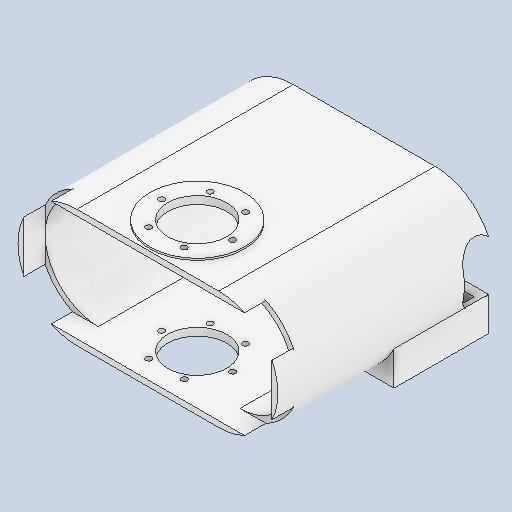
# Autodesk Inventor part: motor_holder_1
Saved by Autodesk Inventor 2025.3 (Build 293356030, 356C)
## iProperties
Created: 2025-09-06
Part Number: motor_holder_1
Material: PLA+ filament
Document SubType Name: Modeling
Designer: MSI
Density: 1.23 g/cm^3
Appearance: 일반
Mass: 781.424 g
Surface Area: 2127.56 cm^2
Volume: 635.304 cm^3
Author: MSI
Autodesk Inventor part; units mm, degrees
ref_plane "YZ Plane" through (0, 0, 0) normal (1, 0, 0) x (0, 1, 0)
ref_plane "XZ Plane" through (0, 0, 0) normal (0, 1, 0) x (-1, 0, 0)
ref_plane "XY Plane" through (0, 0, 0) normal (0, 0, 1) x (1, 0, 0)
sketch "스케치1" plane through (0, 0, 0) normal (0, 0, 1) x (1, 0, 0)
  circle A0 centre (-60, 0) radius 45
  circle A1 centre (60, 0) radius 45
  line L0 (-60, 45) -> (60, 45)
  line L1 (60, -45) -> (-60, -45)
  circle A2 centre (-60, 0) radius 50
  circle A3 centre (60, 0) radius 50
  line L2 (-60, 50) -> (60, 50)
  line L3 (60, -50) -> (-60, -50)
  point P0 (0, 0)
  point P1 (0, 45)
  dimension "d0" = 90
  dimension "d1" = 120
  dimension "d2" = 5
  constraints: 8 end point, 8 point on circle, 8 tangent, 4 centre point, 2 equal radius, 2 horizontal alignment, 1 midpoint, 1 vertical alignment
  measures "d0" diameter of A0
  measures "d1" distance of L1.start L1.end
  measures "d2" radial gap between concentric circles of A0 A2
extrude "돌출1" add sketch "스케치1" along normal mid plane 178 contours A0 L0 A2 L1 | A0 L1 A2 L0 | A2 L2 A3 L0 | L0 A3 L1 A2 | L1 A3 L3 A2 | A3 L1 A1 L0 | L0 A1 L1 A3
sketch "스케치2" plane through (0, 0, -89) normal (0, 0, -1) x (-1, 0, 0)
  arc A0 (-60, 50) -> (-60, -50) centre (-60, 0) ccw projected
  line L0 (-60, -50) -> (60, -50) projected
  arc A1 (60, -50) -> (60, 50) centre (60, 0) ccw projected
  line L1 (60, 50) -> (-60, 50) projected
  circle A2 centre (60, 0) radius 45 projected
  circle A3 centre (-60, 0) radius 45 projected
  point P0 (0, 0)
extrude "돌출2" add sketch "스케치2" along normal blind 5 contours L1 A1 L0 A0 | A2 | A3
sketch "스케치4" plane through (0, 0, 89) normal (0, 0, 1) x (1, 0, 0)
  line L0 (20, 15) -> (-20, 15)
  line L1 (-20, 15) -> (-20, -15)
  line L2 (-20, -15) -> (20, -15)
  line L3 (20, -15) -> (20, 15)
  line L4 (20, 15) -> (-20, -15) construction
  line L5 (-20, 15) -> (20, -15) construction
  point P0 (0, 0)
  dimension "d14" = 40
  dimension "d15" = 30
  constraints: 12 end point, 2 midpoint, 2 parallel, 1 horizontal, 1 perpendicular
  measures "d14" distance of L2.end L1.end
  measures "d15" distance of L1.end L0.end
extrude "돌출4" cut sketch "스케치4" against normal up to surface (178 mm away)
sketch "스케치5" plane through (0, 0, 89) normal (0, 0, 1) x (1, 0, 0)
  arc A0 (17.5736, -15) -> (17.5736, 15) centre (60, 0) ccw projected
  line L0 (-60, 45) -> (60, 45)
  line L1 (60, 45) -> (60, -45)
  line L2 (60, -45) -> (-60, -45)
  line L3 (-60, -45) -> (-60, 45)
  line L4 (-60, 45) -> (60, -45) construction
  line L5 (60, 45) -> (-60, -45) construction
  point P0 (0, 0)
  constraints: 12 end point, 2 midpoint, 2 parallel, 2 tangent, 1 horizontal, 1 perpendicular, 1 point on circle
extrude "돌출5" cut sketch "스케치5" against normal blind 150 contours L2 L3 L0 L1
sketch "스케치6" plane through (0, 0, 89) normal (0, 0, 1) x (1, 0, 0)
  line L0 (105, 45) -> (-105, 45)
  line L1 (-105, 45) -> (-105, -45)
  line L2 (-105, -45) -> (105, -45)
  line L3 (105, -45) -> (105, 45)
  line L4 (105, 45) -> (-105, -45) construction
  line L5 (-105, 45) -> (105, -45) construction
  line L6 (-60, 45) -> (60, 45) projected
  arc A0 (-60, 45) -> (-60, -45) centre (-60, 0) ccw projected
  point P0 (0, 0)
  constraints: 12 end point, 2 midpoint, 2 parallel, 1 collinear, 1 horizontal, 1 perpendicular, 1 tangent
extrude "돌출6" cut sketch "스케치6" against normal blind 18
sketch "스케치3" plane through (0, 0, 0) normal (1, 0, 0) x (0, 1, 0)
  line L0 (10, -84) -> (-10, -84) construction
  line L1 (10, -69) -> (-10, -69)
  line L2 (-10, -99) -> (10, -99)
  arc A0 (10, -99) -> (10, -69) centre (10, -84) ccw
  arc A1 (-10, -69) -> (-10, -99) centre (-10, -84) ccw
  line L3 (-50, -94) -> (50, -94) projected
  point P0 (0, 0)
  point P1 (0, -84)
  dimension "d7" = 10
  dimension "d42" = 15
  constraints: 8 end point, 4 point on circle, 4 tangent, 2 centre point, 1 horizontal, 1 midpoint, 1 parallel, 1 vertical alignment
  measures "d7" distance of point (0, -84) L0.end
  measures "d42" radius of A1
extrude "돌출3" cut sketch "스케치3" along normal through all both and the other way through all
sketch "스케치7" plane through (-60, 50, 89) normal (0, 1, 0) x (1, 0, 0)
  circle A0 centre (60, 41.75) radius 40
  line L0 (0, 183) -> (120, 183) projected
  point P0 (60, 89)
  dimension "d20" = 80
  dimension "d21" = 141.25
  constraints: 1 centre point, 1 vertical alignment
  measures "d20" diameter of A0
  measures "d21" distance from line of L0 A0.centre
extrude "돌출7" add sketch "스케치7" along normal blind 1.5
mirror "미러1" about plane through (0, 0, 0) normal (0, 1, 0) of "돌출7"
sketch "스케치8" plane through (0, 51.5, 47.25) normal (0, 1, 0) x (1, 0, 0)
  circle A0 centre (0, 0) radius 40 projected
  point P0 (0, 47.25)
  constraints: 1 coincident
hole "구멍1" at (0, 51.5, 47.25) direction (0, -1, 0) diameter 50 end through all
sketch "스케치9" plane through (0, 51.5, 47.25) normal (0, 1, 0) x (1, 0, 0)
  circle A0 centre (0, 0) radius 25 construction
  line L0 (0, 0) -> (-30, 0) construction
  point P0 (0, 47.25)
  dimension "d31" = 30
  constraints: 2 end point, 1 coincident, 1 horizontal
  measures "d31" distance of L0.start L0.end
hole "구멍2" at (-30, 51.5, 47.25) direction (0, -1, 0) diameter 5 end through all
pattern_circular "원형 패턴1" count 6 over 360 about axis through (0, -252.6378, 47.25) along (0, 1, 0) of "구멍2"
sketch "스케치10" plane through (0, 0, -94) normal (0, 0, -1) x (-1, 0, 0)
  arc A0 (-105.2923, -21.1803) -> (-60, -50) centre (-60, 0) ccw projected
  line L0 (-105.2923, -21.1803) -> (105.2923, -21.1803)
  line L1 (105.2923, -21.1803) -> (105.2923, -50)
  line L2 (105.2923, -50) -> (-105.2923, -50)
  line L3 (-105.2923, -50) -> (-105.2923, -21.1803)
  line L4 (-60, -50) -> (60, -50) projected
  line L5 (105.2923, -21.1803) -> (-105.2923, -21.1803) projected
  arc A1 (-105.2923, -21.1803) -> (-60, -50) centre (-60, 0) ccw projected
  line L6 (-60, -50) -> (60, -50) projected
  arc A2 (60, -50) -> (105.2923, -21.1803) centre (60, 0) ccw projected
  point P0 (0, 0)
  point P1 (-60, -50)
  constraints: 8 end point, 2 parallel, 1 coincident, 1 collinear, 1 horizontal, 1 perpendicular
extrude "돌출8" add sketch "스케치10" against normal blind 80 contours A0 L2 L3 | L1 L2 A2
sketch "스케치11" plane through (-60, -50, 89) normal (0, -1, 0) x (1, 0, 0)
  line L0 (55, -106.63) -> (65, -106.63)
  line L1 (65, -106.63) -> (65, -179.37)
  line L2 (65, -179.37) -> (55, -179.37)
  line L3 (55, -179.37) -> (55, -106.63)
  line L4 (55, -106.63) -> (65, -179.37) construction
  line L5 (65, -106.63) -> (55, -179.37) construction
  line L6 (-45.2923, -183) -> (-45.2923, -103) projected
  line L7 (55, -106.63) -> (-32.68, -106.63)
  line L8 (-32.68, -106.63) -> (-32.68, -179.37)
  line L9 (-32.68, -179.37) -> (55, -179.37)
  line L10 (55, -179.37) -> (55, -106.63)
  line L11 (65, -106.63) -> (152.68, -106.63)
  line L12 (152.68, -106.63) -> (152.68, -179.37)
  line L13 (152.68, -179.37) -> (65, -179.37)
  line L14 (65, -179.37) -> (65, -106.63)
  point P0 (60, -89)
  point P1 (60, -143)
  point P2 (-45.2923, -143)
  dimension "d45" = 72.74
  dimension "d46" = 10
  dimension "d54" = 87.68
  dimension "d55" = 87.68
  constraints: 28 end point, 6 parallel, 3 horizontal, 3 midpoint, 3 perpendicular, 2 collinear, 1 horizontal alignment, 1 vertical alignment
  measures "d45" distance of L0.end L1.end
  measures "d46" distance of L1.end L2.end
  measures "d54" distance of L8.end L9.end
  measures "d55" distance of L0.end L11.end
hole "구멍3" at (-5, -50, -17.63) at (5, -50, -17.63) at (5, -50, -90.37) at (-5, -50, -90.37) at (-92.68, -50, -17.63) at (-92.68, -50, -90.37) at (92.68, -50, -17.63) at (92.68, -50, -90.37) direction (0, 1, 0) diameter 4 depth 8 tip angle 118
equation "\"d55\" = d54"
